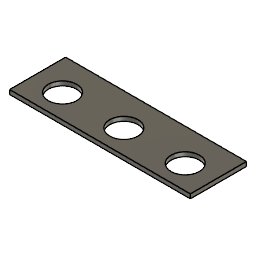
bnc (Autodesk Fusion 360 design; units mm, degrees)
Autodesk Fusion 360 part; units mm, degrees
sketch "Szkic1" plane through (0, 0, 0) normal (0, 0, 1) x (1, 0, 0)
  circle A0 centre (0, 0) radius 6.5
  line L0 (1.75, 0) -> (22.5, 0)
  circle A1 centre (28.2, 0) radius 6.5
  circle A2 centre (56.4, 0) radius 6.5
  line L1 (69.75, -11) -> (-13.35, -11)
  line L2 (-13.35, -11) -> (-13.35, 14.8)
  line L3 (-13.35, 14.8) -> (69.75, 14.8)
  line L4 (69.75, 14.8) -> (69.75, -11)
  point P0 (28.2, 0)
  dimension "d1" = 13
  dimension "d4" = 56.4
  dimension "d5" = 0
  dimension "d6" = 13.35
  dimension "d7" = 11
  dimension "d8" = 14.8
  dimension "d11" = 13.35
  constraint coincident A0.centre origin
  constraint horizontal L1
  constraint perpendicular L1 L2
  constraint parallel L1 L3
  constraint parallel L2 L4
  constraint coincident P0 A1.centre
  measures "d1" diameter of A0
  measures "d6" distance of A0.centre L2
  measures "d7" distance of A0.centre L1
  measures "d8" distance of A0.centre L3
  measures "d11" distance of A2.centre L4
extrude "Wyciągnięcie proste1" add sketch "Szkic1" along normal blind 2
equation "d4 = ( 28.2 * 2 ) * 1 mm"
